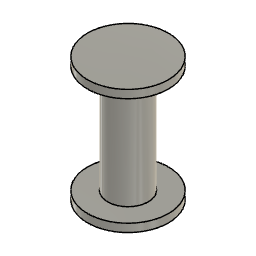
Assembly_2 v1 (Autodesk Fusion 360 archive; units mm, degrees)
design "Motor"
Autodesk Fusion 360 part; units mm, degrees
sketch "Schizzo1" plane through (0, 0, 0) normal (0, 0, 1) x (1, 0, 0)
  circle A0 centre (0, 0) radius 75
  dimension "d1" = 150
  constraint coincident A0.centre origin
  measures "d1" diameter of A0
extrude "Estrusione1" add sketch "Schizzo1" along normal mid plane 400
sketch "Schizzo2" plane through (0, 0, 0) normal (0, 0, 1) x (1, 0, 0)
  circle A0 centre (0, 0) radius 150
  dimension "d4" = 300
  constraint coincident A0.centre origin
  measures "d4" diameter of A0
extrude "Estrusione2" add sketch "Schizzo2" along normal blind 30 from surface at 200
extrude "Estrusione3" add 1 faces at (124.4415, -7.4521, 200) along direction (0, 0, -1) blind 30 from surface at 400
extrude "Estrusione4" add sketch "Schizzo1" against normal blind 30 from surface at -200

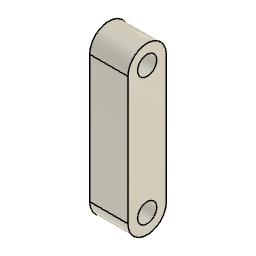
design "Link1"
Autodesk Fusion 360 part; units mm, degrees
sketch "Schizzo3" plane through (0, 0, 0) normal (0, 0, 1) x (1, 0, 0)
  line L0 (0, -150) -> (1000, -150)
  line L1 (0, 150) -> (1000, 150)
  arc A0 (1000, -150) -> (1000, 150) centre (1000, 0) ccw
  arc A1 (0, 150) -> (0, -150) centre (0, 0) ccw
  dimension "d5" = 1000
  dimension "d6" = 1000
  constraint coincident A1.centre origin
  constraint horizontal L0
  constraint horizontal L1
  constraint tangent L1 A0
  measures "d5" distance of L0.start L0.end
  measures "d6" distance of L1.start L1.end
extrude "Estrusione2" add sketch "Schizzo3" along normal mid plane 300
sketch "Schizzo4" plane through (0, 0, 150) normal (0, 0, 1) x (-1, 0, 0)
  arc A0 (0, -150) -> (0, 150) centre (0, 0) ccw
  line L0 (0, 150) -> (-1000, 150)
  arc A1 (-1000, 150) -> (-1000, -150) centre (-1000, 0) ccw
  line L1 (-1000, -150) -> (0, -150)
  circle A2 centre (0, 0) radius 75
  dimension "d9" = 150
  constraint concentric A0 A2
  measures "d9" diameter of A2
extrude "Estrusione3" cut sketch "Schizzo4" along normal through all and the other way through all contours A2
sketch "Schizzo5" plane through (0, 0, 0) normal (0, 0, 1) x (1, 0, 0)
  circle A0 centre (1000, 0) radius 75
  dimension "d11" = 150
  measures "d11" diameter of A0
extrude "Estrusione4" cut sketch "Schizzo5" along normal through all and the other way through all
move_body "Sposta1" bodies 1 to x (0, 0, 1) y (0, 1, 0) z (-1, 0, 0) at (0, 0, 0)

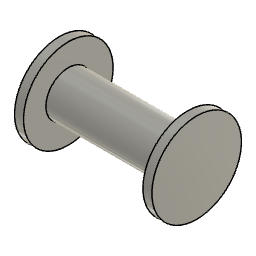
design "Motor_prismatic"
Autodesk Fusion 360 part; units mm, degrees
sketch "Schizzo1" plane through (0, 0, 0) normal (0, 0, 1) x (1, 0, 0)
  circle A0 centre (0, 0) radius 75
  dimension "d1" = 150
  constraint coincident A0.centre origin
  measures "d1" diameter of A0
extrude "Estrusione1" add sketch "Schizzo1" along normal mid plane 400
sketch "Schizzo2" plane through (0, 0, 0) normal (0, 0, 1) x (1, 0, 0)
  circle A0 centre (0, 0) radius 150
  dimension "d4" = 300
  constraint coincident A0.centre origin
  measures "d4" diameter of A0
extrude "Estrusione2" add sketch "Schizzo2" along normal blind 30 from surface at 200
extrude "Estrusione3" add 1 faces at (124.4415, -7.4521, 200) along direction (0, 0, -1) blind 30 from surface at 400
extrude "Estrusione4" add sketch "Schizzo1" against normal blind 30 from surface at -200
move_body "Sposta1" bodies 1 to x (0, 0, 1) y (0, 1, 0) z (-1, 0, 0) at (0, 0, 0)

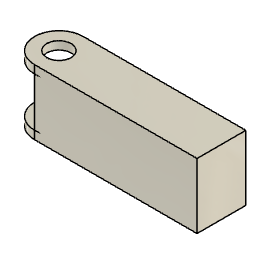
design "Link2"
Autodesk Fusion 360 part; units mm, degrees
sketch "Schizzo1" plane through (0, 0, 0) normal (0, 0, 1) x (1, 0, 0)
  line L0 (150, 0) -> (150, 1000)
  line L1 (-150, 1000) -> (-150, 0)
  arc A0 (-150, 0) -> (150, 0) centre (0, 0) ccw
  line L2 (150, 1000) -> (-150, 1000)
  dimension "d1" = 300
  dimension "d2" = 1000
  constraint coincident A0.centre origin
  constraint vertical L0
  constraint tangent L1 A0
  constraint vertical L1
  constraint perpendicular L1 L2
  measures "d1" diameter of A0
  measures "d2" distance of L0.start L0.end
sketch "Schizzo2" plane through (0, 0, 0) normal (0, 0, 1) x (1, 0, 0)
  circle A0 centre (0, 0) radius 150
  dimension "d6" = 300
  constraint coincident A0.centre origin
  measures "d6" diameter of A0
sketch "Schizzo3" plane through (0, 0, 0) normal (0, 0, 1) x (1, 0, 0)
sketch "Schizzo4" plane through (0, 0, 0) normal (0, 0, 1) x (1, 0, 0)
  line L0 (0, -150) -> (1000, -150)
  line L1 (0, 150) -> (1000, 150)
  line L2 (1000, 150) -> (1000, -150)
  arc A0 (0, 150) -> (0, -150) centre (0, 0) ccw
  dimension "d10" = 300
  dimension "d11" = 1000
  dimension "d12" = 1000
  constraint coincident A0.centre origin
  constraint horizontal L0
  constraint horizontal L1
  constraint perpendicular L0 L2
  measures "d10" diameter of A0
  measures "d11" distance of L0.start L0.end
  measures "d12" distance of L1.start L1.end
extrude "Estrusione3" add sketch "Schizzo4" along normal mid plane 400
sketch "Schizzo5" plane through (0, 0, 0) normal (0, 0, 1) x (1, 0, 0)
  circle A0 centre (0, 0) radius 150
  dimension "d15" = 300
  constraint coincident A0.centre origin
  measures "d15" diameter of A0
extrude "Estrusione4" cut sketch "Schizzo5" along normal mid plane 300
sketch "Schizzo6" plane through (0, 0, 0) normal (0, 0, 1) x (1, 0, 0)
  circle A0 centre (0, 0) radius 75
  dimension "d18" = 150
  constraint coincident A0.centre origin
  measures "d18" diameter of A0
extrude "Estrusione5" cut sketch "Schizzo6" along normal through all and the other way through all

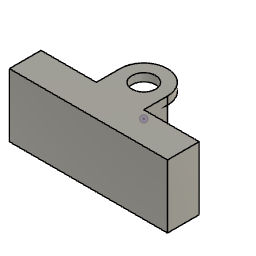
design "Basis"
Autodesk Fusion 360 part; units mm, degrees
sketch "Schizzo1" plane through (0, 0, 0) normal (0, 0, 1) x (1, 0, 0)
sketch "Schizzo2" plane through (0, 0, 0) normal (0, 0, 1) x (1, 0, 0)
  line L0 (150, 0) -> (150, -150)
  line L1 (150, -150) -> (500, -150)
  line L2 (500, -150) -> (500, -350)
  line L3 (500, -350) -> (-500, -350)
  line L4 (-500, -350) -> (-500, -150)
  line L5 (-500, -150) -> (-150, -150)
  line L6 (-150, -150) -> (-150, 0)
  arc A0 (150, 0) -> (-150, 0) centre (0, 0) ccw
  dimension "d7" = 300
  dimension "d8" = 150
  constraint coincident A0.centre origin
  constraint vertical L0
  constraint perpendicular L0 L1
  constraint perpendicular L1 L2
  constraint perpendicular L2 L3
  constraint perpendicular L1 L4
  constraint perpendicular L4 L5
  constraint perpendicular L5 L6
  measures "d7" diameter of A0
  measures "d8" distance of L0.start L0.end
extrude "Estrusione1" add sketch "Schizzo2" along normal mid plane 400
ref_plane "Piano di lavoro1" through (0, -100, 0) normal (0, 0, 1) x (1, 0, 0)
sketch "Schizzo3" plane through (0, -100, 0) normal (0, 0, 1) x (1, 0, 0)
  circle A0 centre (0, 100) radius 150
  dimension "d11" = 300
  measures "d11" diameter of A0
extrude "Estrusione2" cut sketch "Schizzo3" along normal mid plane 300
sketch "Schizzo4" plane through (0, 0, 0) normal (0, 0, 1) x (1, 0, 0)
  circle A0 centre (0, 0) radius 75
  dimension "d14" = 150
  constraint coincident A0.centre origin
  measures "d14" diameter of A0
extrude "Estrusione3" cut sketch "Schizzo4" along normal through all and the other way through all
